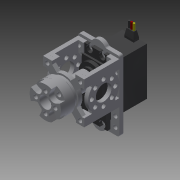
# Autodesk Inventor part: Servo with servo blocks
Saved by Autodesk Inventor 2013 (Build 170138000, 138)
## iProperties
Created: 2012-11-17
Part Number: Servo with servo blocks
Material: Generic
Document SubType Name: Modeling
Designer: niemitalo_dan
Density: 1 g/cm^3
Author: niemitalo_dan
Autodesk Inventor part; units mm, degrees
ref_plane "YZ Plane" through (0, 0, 0) normal (1, 0, 0) x (0, 1, 0)
ref_plane "XZ Plane" through (0, 0, 0) normal (0, 1, 0) x (-1, 0, 0)
sketch "Sketch1" plane through (0, 0, 0) normal (0, 0, 1) x (1, 0, 0)
  line L0 (-9.9314, 19.3675) -> (9.9314, 19.3675)
  line L1 (9.9314, 19.3675) -> (9.9314, -19.3675)
  line L2 (9.9314, -19.3675) -> (-9.9314, -19.3675)
  line L3 (-9.9314, -19.3675) -> (-9.9314, 19.3675)
  point P0 (0, 0)
  point P1 (-9.9314, 0)
  point P2 (0, 19.3675)
  dimension "d0" = 19.8628
  dimension "d1" = 38.735
  constraints: 8 end point, 2 midpoint, 2 parallel, 1 horizontal, 1 horizontal alignment, 1 perpendicular, 1 vertical alignment
  measures "d0" distance of L1.end L2.end
  measures "d1" distance of L0.end L1.end
extrude "Extrusion1" add sketch "Sketch1" along normal blind 33.147
sketch "Sketch2" plane through (0, 0, 33.147) normal (0, 0, 1) x (1, 0, 0)
  line L0 (9.9314, 19.3675) -> (-9.9314, 19.3675) projected
  line L1 (-9.9314, 19.3675) -> (-9.9314, -19.3675) projected
  line L2 (-9.9314, -19.3675) -> (9.9314, -19.3675) projected
  line L3 (-9.2964, 18.7325) -> (9.2964, 18.7325)
  line L4 (9.2964, 18.7325) -> (9.2964, -15.0495)
  line L5 (9.2964, -15.0495) -> (-9.2964, -15.0495)
  line L6 (-9.2964, -15.0495) -> (-9.2964, 18.7325)
  arc A0 (-3.6998, -15.0495) -> (3.6998, -15.0495) centre (0, -10.9617) ccw
  point P0 (0, 0)
  point P1 (0, 18.7325)
  dimension "d4" = 0.635
  dimension "d5" = 0.635
  dimension "d6" = 4.318
  constraints: 8 end point, 2 parallel, 2 point on circle, 2 point on line, 2 vertical alignment, 1 centre point, 1 horizontal, 1 midpoint, 1 perpendicular
  measures "d4" distance between parallel lines of L0 L3
  measures "d5" distance between parallel lines of L1 L6
  measures "d6" distance between parallel lines of L2 L5
extrude "Extrusion2" add sketch "Sketch2" along normal blind 2.794 contours L3 L4 L5 L6
sketch "Sketch3" plane through (0, 0, 35.941) normal (0, 0, 1) x (1, 0, 0)
  circle A0 centre (0, 9.4361) radius 6.4516
  line L0 (9.9314, 19.3675) -> (-9.9314, 19.3675) projected
  point P0 (0, 0)
  dimension "d9" = 12.9032
  dimension "d11" = 9.9314
  constraints: 1 centre point, 1 vertical alignment
  measures "d9" diameter of A0
  measures "d11" distance from line of L0 A0.centre
extrude "Extrusion3" add sketch "Sketch3" along normal blind 1.778
fillet "Fillet1" radius 9.2964 2 edges at (9.2964, 18.7325, 34.544) (-9.2964, 18.7325, 34.544)
ref_plane "Work Plane1" through (0, 0, 29.083) normal (0, 0, 1) x (1, 0, 0)
sketch "Sketch4" plane through (0, 0, 29.083) normal (0, 0, 1) x (1, 0, 0)
  line L0 (9.9314, 19.3675) -> (9.9314, -19.3675) projected
  line L1 (9.9314, -19.3675) -> (-9.9314, -19.3675) projected
  line L2 (-9.9314, -19.3675) -> (-9.9314, 19.3675) projected
  line L3 (-9.9314, 19.3675) -> (9.9314, 19.3675) projected
  line L4 (-9.3599, 19.3675) -> (9.3599, 19.3675)
  line L5 (9.3599, 19.3675) -> (9.3599, 26.4795)
  line L6 (-9.3599, 26.4795) -> (-9.3599, 19.3675)
  circle A0 centre (-5.1689, 23.9395) radius 2.667
  circle A1 centre (5.1689, 23.9395) radius 2.667
  line L7 (-5.9821, 26.4795) -> (-9.3599, 26.4795)
  line L8 (9.3599, 26.4795) -> (5.9821, 26.4795)
  line L9 (4.3557, 26.4795) -> (-4.3557, 26.4795)
  point P0 (0, 0)
  point P1 (0, 26.4795)
  dimension "d16" = 18.7198
  dimension "d18" = 7.112
  dimension "d20" = 5.334
  dimension "d21" = 4.191
  dimension "d22" = 4.191
  constraints: 12 end point, 4 parallel, 4 point on circle, 2 centre point, 1 equal radius, 1 horizontal, 1 horizontal alignment, 1 midpoint, 1 perpendicular, 1 point on line, 1 vertical alignment
  measures "d16" distance of L5.end L6.start
  measures "d18" distance of L6.start L4.start
  measures "d20" diameter of A0
  measures "d21" distance from line of L6 A0.centre
  measures "d22" distance from line of L5 A1.centre
extrude "Extrusion4" add sketch "Sketch4" along normal blind 2.54 contours L3 L6 L7 A0 L9 A1 L8 L5
fillet "Fillet2" radius 0.254 4 edges at (-5.9821, 26.4795, 30.353) (-4.3557, 26.4795, 30.353) (4.3557, 26.4795, 30.353) (5.9821, 26.4795, 30.353)
mirror "Mirror1" about plane through (0, 0, 0) normal (0, 1, 0) of "Extrusion4", "Fillet2"
sketch "Sketch5" plane through (-9.9314, 19.3675, 0) normal (0, 1, 0) x (1, 0, 0)
  line L0 (0, 0) -> (19.8628, 0) projected
  line L1 (6.1214, -0.254) -> (13.7414, -0.254)
  line L2 (13.7414, -0.254) -> (13.7414, -4.572)
  line L3 (13.7414, -4.572) -> (6.1214, -4.572)
  line L4 (6.1214, -4.572) -> (6.1214, -0.254)
  point P0 (9.9314, 0)
  point P1 (9.9314, -0.254)
  point P2 (9.9314, 0)
  dimension "d26" = 7.62
  dimension "d27" = 4.318
  dimension "d28" = 0.254
  constraints: 8 end point, 2 midpoint, 2 parallel, 1 horizontal, 1 perpendicular, 1 vertical alignment
  measures "d26" distance of L2.end L3.end
  measures "d27" distance of L1.end L2.end
  measures "d28" distance between parallel lines of L0 L1
extrude "Extrusion5" add sketch "Sketch5" along normal blind 1.5875
sketch "Sketch6" plane through (-9.9314, 20.955, 0) normal (0, 1, 0) x (1, 0, 0)
  line L0 (13.7414, -0.254) -> (6.1214, -0.254) projected
  line L1 (6.1214, -0.254) -> (6.1214, -4.572) projected
  line L2 (6.1214, -4.572) -> (13.7414, -4.572) projected
  line L3 (13.7414, -4.572) -> (13.7414, -0.254) projected
  point P0 (9.9314, 0)
extrude "Extrusion6" add sketch "Sketch6" along normal blind 5.08 draft -10
sketch "Sketch7" plane through (-9.9314, 26.035, 0) normal (0, 1, 0) x (1, 0, 0)
  circle A0 centre (9.9314, -2.413) radius 0.7937
  point P0 (9.9314, 0)
  dimension "d33" = 1.5875
  constraints: 1 centre point
  measures "d33" diameter of A0
extrude "Extrusion7" add sketch "Sketch7" along normal blind 5.08 separate body
sketch "Sketch8" plane through (-9.9314, 26.035, 0) normal (0, 1, 0) x (1, 0, 0)
  line L0 (7.0171, -3.6763) -> (7.0171, -1.1497) projected
  circle A0 centre (8.0331, -2.413) radius 0.7937
  point P0 (9.9314, 0)
  dimension "d36" = 1.5875
  dimension "d37" = 1.016
  constraints: 1 centre point
  measures "d36" diameter of A0
  measures "d37" distance from line of L0 A0.centre
extrude "Extrusion8" add sketch "Sketch8" along normal blind 5.08 bodies 1
sketch "Sketch9" plane through (-9.9314, 26.035, 0) normal (0, 1, 0) x (1, 0, 0)
  line L0 (12.8457, -1.1497) -> (12.8457, -3.6763) projected
  circle A0 centre (11.8297, -2.413) radius 0.7938
  point P0 (9.9314, 0)
  dimension "d40" = 1.5875
  dimension "d41" = 1.016
  constraints: 1 centre point
  measures "d40" diameter of A0
  measures "d41" distance from line of L0 A0.centre
extrude "Extrusion9" add sketch "Sketch9" along normal blind 5.08 separate body
sketch "Sketch10" plane through (0, 0, 29.083) normal (0, 0, -1) x (-1, 0, 0)
  line L0 (-9.9314, -19.3675) -> (-9.9314, 19.3675) construction
  line L1 (-9.9314, 19.3675) -> (-9.3599, 19.3675) construction
  line L2 (-9.3599, 19.3675) -> (-9.3599, 26.4795) construction
  line L3 (-9.3599, 26.4795) -> (-6.9873, 26.4795) construction
  arc A0 (-6.8291, 26.0267) -> (-6.9873, 26.4795) centre (-6.9873, 26.2255) ccw construction
  arc A1 (-6.8291, 26.0267) -> (-3.5087, 26.0267) centre (-5.1689, 23.9395) ccw construction
  arc A2 (-3.3505, 26.4795) -> (-3.5087, 26.0267) centre (-3.3505, 26.2255) ccw construction
  line L4 (-3.3505, 26.4795) -> (3.3505, 26.4795) construction
  arc A3 (3.5087, 26.0267) -> (3.3505, 26.4795) centre (3.3505, 26.2255) ccw construction
  arc A4 (3.5087, 26.0267) -> (6.8291, 26.0267) centre (5.1689, 23.9395) ccw construction
  arc A5 (6.9873, 26.4795) -> (6.8291, 26.0267) centre (6.9873, 26.2255) ccw construction
  line L5 (6.9873, 26.4795) -> (9.3599, 26.4795) construction
  line L6 (9.3599, 26.4795) -> (9.3599, 19.3675) construction
  line L7 (9.3599, 19.3675) -> (9.9314, 19.3675) construction
  line L8 (9.9314, 19.3675) -> (9.9314, -19.3675) construction
  line L9 (9.9314, -19.3675) -> (9.3599, -19.3675) construction
  line L10 (9.3599, -19.3675) -> (-9.3599, -19.3675) construction
  line L11 (-9.3599, -19.3675) -> (-9.9314, -19.3675) construction
  line L12 (-9.3599, 19.3675) -> (9.3599, 19.3675) construction
  line L13 (9.3599, -19.3675) -> (9.3599, -26.4795) construction
  line L14 (9.3599, -26.4795) -> (6.9873, -26.4795) construction
  arc A6 (6.8291, -26.0267) -> (6.9873, -26.4795) centre (6.9873, -26.2255) ccw construction
  arc A7 (6.8291, -26.0267) -> (3.5087, -26.0267) centre (5.1689, -23.9395) ccw construction
  arc A8 (3.3505, -26.4795) -> (3.5087, -26.0267) centre (3.3505, -26.2255) ccw construction
  line L15 (3.3505, -26.4795) -> (-3.3505, -26.4795) construction
  arc A9 (-3.5087, -26.0267) -> (-3.3505, -26.4795) centre (-3.3505, -26.2255) ccw construction
  arc A10 (-3.5087, -26.0267) -> (-6.8291, -26.0267) centre (-5.1689, -23.9395) ccw construction
  arc A11 (-6.9873, -26.4795) -> (-6.8291, -26.0267) centre (-6.9873, -26.2255) ccw construction
  line L16 (-6.9873, -26.4795) -> (-9.3599, -26.4795) construction
  line L17 (-9.3599, -26.4795) -> (-9.3599, -19.3675) construction
  line L18 (-16.6688, 28.575) -> (16.6687, 28.575)
  line L19 (16.6687, 28.575) -> (16.6688, -28.575)
  line L20 (16.6688, -28.575) -> (-16.6687, -28.575)
  line L21 (-16.6687, -28.575) -> (-16.6688, 28.575)
  line L22 (-9.9314, 19.3675) -> (9.9314, 19.3675)
  line L23 (9.9314, 19.3675) -> (9.9314, -19.3675)
  line L24 (9.9314, -19.3675) -> (-9.9314, -19.3675)
  line L25 (-9.9314, -19.3675) -> (-9.9314, 19.3675)
  circle A12 centre (-5.1689, 23.9395) radius 1.7272
  circle A13 centre (5.1689, 23.9395) radius 1.7272
  circle A14 centre (-5.1689, -23.9395) radius 1.7272
  circle A15 centre (5.1689, -23.9395) radius 1.7272
  circle A16 centre (-13.3033, 23.075) radius 1.7272
  arc A17 (5.4993, 28.575) -> (-5.4993, 28.575) centre (0, 25.4) ccw
  line L26 (-21.6347, 31.75) -> (28.9033, 31.75) construction
  arc A18 (-5.4993, -28.575) -> (5.4993, -28.575) centre (0, -25.4) ccw
  line L27 (-14.4215, -31.75) -> (20.7079, -31.75) construction
  circle A19 centre (13.3033, 23.075) radius 1.7272
  circle A20 centre (-13.3033, 15.1375) radius 1.7272
  circle A21 centre (-13.3033, 4.0885) radius 1.7272
  circle A22 centre (13.3032, 15.1375) radius 1.7272
  circle A23 centre (13.3032, 4.0885) radius 1.7272
  line L28 (-16.6688, 0) -> (16.6688, 0) construction
  circle A24 centre (-13.3033, -23.075) radius 1.7272
  circle A25 centre (13.3033, -23.075) radius 1.7272
  circle A26 centre (-13.3033, -15.1375) radius 1.7272
  circle A27 centre (-13.3033, -4.0885) radius 1.7272
  circle A28 centre (13.3032, -15.1375) radius 1.7272
  circle A29 centre (13.3032, -4.0885) radius 1.7272
  point P0 (0, 0)
  point P1 (0, 28.575)
  dimension "d44" = 3.4544
  dimension "d47" = 57.15
  dimension "d48" = 3.175
  dimension "d49" = 6.35
  dimension "d50" = 6.35
  dimension "d51" = 3.175
  dimension "d52" = 5.5
  dimension "d53" = 3.3655
  dimension "d54" = 3.3655
  dimension "d55" = 33.3375
  dimension "d56" = 7.9375
  dimension "d57" = 11.049
  constraints: 22 end point, 18 centre point, 9 equal radius, 7 vertical alignment, 6 symmetric about line, 5 parallel, 4 coincident, 4 horizontal alignment, 4 point on circle, 4 point on line, 3 midpoint, 3 perpendicular, 2 horizontal, 2 tangent, 6 other
  measures "d44" diameter of A12
  measures "d47" distance of L20.end L18.start
  measures "d48" distance between parallel lines of L18 L26
  measures "d49" radius of A17
  measures "d50" radius of A18
  measures "d51" distance between parallel lines of L20 L27
  measures "d52" distance from line of L18 A16.centre
  measures "d53" distance from line of L21 A16.centre
  measures "d54" distance from line of L19 A19.centre
  measures "d55" distance of L19.end L20.end
  measures "d56" distance of A16.centre A20.centre
  measures "d57" distance of A20.centre A21.centre
extrude "Extrusion10" add sketch "Sketch10" along normal blind 3.175 separate body
fillet "Fillet3" radius 1.5875 8 edges at (-16.6687, 28.575, 27.4955) (-16.6688, -28.575, 27.4955) (-5.4993, -28.575, 27.4955) (5.4993, -28.575, 27.4955) (16.6687, -28.575, 27.4955) (5.4993, 28.575, 27.4955) (16.6688, 28.575, 27.4955) (-5.4993, 28.575, 27.4955)
sketch "Sketch11" plane through (0, 9.4361, 37.719) normal (0, 0, 1) x (1, 0, 0)
  circle A0 centre (0, 0) radius 6.4516 projected
  circle A1 centre (0, 0) radius 1.5875
  point P0 (0, -9.4361)
  dimension "d61" = 3.175
  constraints: 1 centre point, 1 coincident
  measures "d61" diameter of A1
extrude "Extrusion11" add sketch "Sketch11" along normal blind 1.5875 separate body contours A1
sketch "Sketch12" plane through (0, 0, 29.083) normal (0, 0, 1) x (1, 0, 0)
  line L0 (-9.9314, -19.3675) -> (-9.9314, 19.3675) projected
  line L1 (-9.9314, 19.3675) -> (9.9314, 19.3675) projected
  line L2 (9.9314, 19.3675) -> (9.9314, -19.3675) projected
  circle A0 centre (-13.3032, -4.0885) radius 1.7272 projected
  circle A1 centre (13.3033, -4.0885) radius 1.7272 projected
  circle A2 centre (-13.3033, 23.075) radius 1.7272 projected
  circle A3 centre (13.3033, 23.075) radius 1.7272 projected
  line L3 (6.35, 28.575) -> (15.0813, 28.575) projected
  line L4 (-15.0812, 28.575) -> (-6.35, 28.575) projected
  line L5 (-16.6688, -26.9875) -> (-16.6687, 26.9875) projected
  line L6 (16.6688, 26.9875) -> (16.6687, -26.9875) projected
  line L7 (-16.6687, 26.4668) -> (-9.3918, 26.4668)
  line L8 (-9.3918, 26.4668) -> (-9.3918, 19.3675)
  line L9 (-9.3918, 19.3675) -> (-16.6687, 19.3675)
  line L10 (-16.6687, 19.3675) -> (-16.6687, 26.4668)
  line L11 (-16.6688, -0.9135) -> (-9.9314, -0.9135)
  line L12 (-9.9314, -0.9135) -> (-9.9314, -7.2635)
  line L13 (-9.9314, -7.2635) -> (-16.6688, -7.2635)
  line L14 (-16.6688, -7.2635) -> (-16.6688, -0.9135)
  line L15 (16.6688, -0.9135) -> (9.9314, -0.9135)
  line L16 (9.9314, -0.9135) -> (9.9314, -7.2635)
  line L17 (9.9314, -7.2635) -> (16.6688, -7.2635)
  line L18 (16.6688, -7.2635) -> (16.6688, -0.9135)
  line L19 (9.3087, 19.3675) -> (16.6688, 19.3675)
  line L20 (16.6688, 19.3675) -> (16.6688, 26.4668)
  line L21 (16.6688, 26.4668) -> (9.3087, 26.4668)
  line L22 (9.3087, 26.4668) -> (9.3087, 19.3675)
  point P0 (0, 0)
  dimension "d66" = 2.1082
  dimension "d67" = 2.1082
  dimension "d68" = 3.175
  dimension "d69" = 3.175
  constraints: 32 end point, 8 parallel, 8 point on line, 4 horizontal, 4 perpendicular, 2 collinear
  measures "d66" distance between parallel lines of L4 L7
  measures "d67" distance between parallel lines of L3 L21
  measures "d68" distance from line of L11 A0.centre
  measures "d69" distance from line of L13 A0.centre
extrude "Extrusion12" add sketch "Sketch12" along normal blind 3.175 separate body contours L13 L5 L11 L0 | L9 L5 L7 L8 L1
sketch "Sketch13" plane through (0, 0, 32.258) normal (0, 0, 1) x (1, 0, 0)
  line L0 (-16.6687, 26.4668) -> (-13.4937, 26.4668)
  line L1 (-13.4937, 26.4668) -> (-13.4937, -7.2635)
  line L2 (-13.4937, -7.2635) -> (-16.6687, -7.2635)
  line L3 (-16.6687, -7.2635) -> (-16.6687, 26.4668)
  line L4 (9.9314, 19.3675) -> (9.9314, -19.3675) projected
  line L5 (9.9314, -19.3675) -> (-9.9314, -19.3675) projected
  line L6 (-9.9314, -19.3675) -> (-9.9314, 19.3675) projected
  line L7 (-9.9314, 19.3675) -> (9.9314, 19.3675) projected
  circle A0 centre (-13.3033, 23.075) radius 1.7272 projected
  line L8 (-9.3918, 19.3675) -> (-16.6687, 19.3675) projected
  line L9 (-16.6687, 19.3675) -> (-16.6687, 26.4668) projected
  line L10 (-16.6687, 26.4668) -> (-9.3918, 26.4668) projected
  line L11 (-9.3918, 26.4668) -> (-9.3918, 19.3675) projected
  circle A1 centre (-13.3032, -4.0885) radius 1.7272 projected
  line L12 (-16.6688, -0.9135) -> (-9.9314, -0.9135) projected
  line L13 (-9.9314, -0.9135) -> (-9.9314, -7.2635) projected
  line L14 (-9.9314, -7.2635) -> (-16.6688, -7.2635) projected
  line L15 (-16.6688, -7.2635) -> (-16.6688, -0.9135) projected
  line L16 (-16.6688, -7.2635) -> (-9.9314, -7.2635) projected
  point P0 (0, 0)
  dimension "d72" = 3.175
  constraints: 8 end point, 2 parallel, 1 collinear, 1 horizontal, 1 perpendicular
  measures "d72" distance of L1.end L2.end
extrude "Extrusion13" add sketch "Sketch13" along normal blind 19.05 contours L0 L1 A0 L8 L3 | L8 L1 L12 L3 | L1 A0 | L12 L1 A1 L2 L3 | L1 A1 picked at (-13.6297, 22.5349) picked at (-13.989, -3.9498) bodies 6
sketch "Sketch14" plane through (0, 0, 51.308) normal (0, 0, 1) x (1, 0, 0)
  line L0 (-13.4937, 26.4668) -> (-13.4937, 24.7917) construction
  arc A0 (-13.4937, 21.3583) -> (-13.4937, 24.7917) centre (-13.3033, 23.075) ccw construction
  line L1 (-13.4937, 21.3583) -> (-13.4937, 19.3675) construction
  line L2 (-13.4937, 19.3675) -> (-9.3918, 19.3675) construction
  line L3 (-9.3918, 19.3675) -> (-9.3918, 26.4668) construction
  line L4 (-9.3918, 26.4668) -> (-13.4937, 26.4668) construction
  line L5 (-13.4937, -0.9135) -> (-13.4937, -2.3718) construction
  arc A1 (-13.4937, -5.8052) -> (-13.4937, -2.3718) centre (-13.3032, -4.0885) ccw construction
  line L6 (-13.4937, -5.8052) -> (-13.4937, -7.2635) construction
  line L7 (-13.4937, -7.2635) -> (-9.9314, -7.2635) construction
  line L8 (-9.9314, -7.2635) -> (-9.9314, -0.9135) construction
  line L9 (-9.9314, -0.9135) -> (-13.4937, -0.9135) construction
  line L10 (-16.6687, 19.3675) -> (-13.4937, 19.3675) construction
  line L11 (-13.4937, -0.9135) -> (-16.6688, -0.9135) construction
  circle A2 centre (-13.3033, 23.075) radius 1.7272 construction
  circle A3 centre (-13.3032, -4.0885) radius 1.7272 construction
  line L12 (-16.6687, 26.4668) -> (-9.3918, 26.4668)
  line L13 (-9.3918, 26.4668) -> (-9.3918, 19.3675)
  line L14 (-9.3918, 19.3675) -> (-16.6687, 19.3675)
  line L15 (-16.6687, 19.3675) -> (-16.6687, 26.4668)
  line L16 (-16.6688, -0.9135) -> (-9.9314, -0.9135)
  line L17 (-9.9314, -0.9135) -> (-9.9314, -7.2635)
  line L18 (-9.9314, -7.2635) -> (-16.6688, -7.2635)
  line L19 (-16.6688, -7.2635) -> (-16.6688, -0.9135)
  circle A4 centre (-13.3032, -4.0885) radius 1.7272
  circle A5 centre (-13.3033, 23.075) radius 1.7272
  point P0 (0, 0)
  constraints: 16 end point, 4 parallel, 2 centre point, 2 coincident, 2 horizontal, 2 perpendicular, 1 concentric
extrude "Extrusion14" add sketch "Sketch14" along normal blind 3.175 bodies 6
sketch "Sketch16" plane through (-16.6688, 19.3675, 29.083) normal (-1, 0, 0) x (0, 0, 1)
  line L0 (22.225, 0) -> (22.225, -20.281) projected
  line L1 (0, 7.0993) -> (25.4, 7.0993) projected
  line L2 (3.175, 0) -> (3.175, -20.281) projected
  circle A0 centre (12.7, -10.1405) radius 12.7
  line L3 (3.175, -1.7402) -> (3.175, -18.5408)
  line L4 (22.225, -1.7402) -> (22.225, -18.5408)
  point P0 (-29.083, -19.3675)
  point P1 (12.7, 7.0993)
  point P2 (22.225, -10.1405)
  dimension "d80" = 25.4
  constraints: 4 end point, 4 point on circle, 4 point on line, 2 midpoint, 1 centre point, 1 horizontal alignment, 1 vertical alignment
  measures "d80" diameter of A0
extrude "Extrusion15" add sketch "Sketch16" against normal blind 3.175 contours A0 L0 | L2 A0 bodies 6
sketch "Sketch17" plane through (-16.6688, 19.3675, 29.083) normal (-1, 0, 0) x (0, 0, 1)
  arc A0 (22.225, -18.5408) -> (22.225, -1.7402) centre (12.7, -10.1405) ccw construction
  arc A1 (3.175, -1.7402) -> (3.175, -18.5408) centre (12.7, -10.1405) ccw construction
  circle A2 centre (12.7, -10.1405) radius 6.35
  circle A3 centre (12.7, -10.1405) radius 9.525 construction
  circle A4 centre (12.7, -0.6155) radius 1.7272
  circle A5 centre (5.9648, -3.4053) radius 1.7272
  circle A6 centre (3.175, -10.1405) radius 1.7272
  circle A7 centre (5.9648, -16.8757) radius 1.7272
  circle A8 centre (12.7, -19.6655) radius 1.7272
  circle A9 centre (19.4352, -16.8757) radius 1.7272
  circle A10 centre (22.225, -10.1405) radius 1.7272
  circle A11 centre (19.4352, -3.4053) radius 1.7272
  point P0 (-29.083, -19.3675)
  dimension "d85" = 19.05
  dimension "d84" = 12.7
  dimension "d86" = 3.4544
  dimension "d89" = 360
  constraints: 9 centre point, 2 coincident, 2 vertical alignment, 19 other
  measures "d84" diameter of A2
  measures "d86" diameter of A4
extrude "Extrusion16" cut sketch "Sketch17" against normal blind 3.175 bodies 6
mirror "Mirror2" about plane through (0, 0, 0) normal (1, 0, 0) bodies 6
sketch "Sketch18" plane through (0, 0, 54.483) normal (0, 0, 1) x (1, 0, 0)
  circle A0 centre (-13.3033, 23.075) radius 1.7272 projected
  line L0 (-16.6687, 19.3675) -> (-9.3918, 19.3675) projected
  line L1 (-9.3918, 19.3675) -> (-9.3918, 26.4668) projected
  circle A1 centre (-13.3032, -4.0885) radius 1.7272 projected
  line L2 (-9.9314, -7.2635) -> (-9.9314, -0.9135) projected
  line L3 (-9.9314, -0.9135) -> (-16.6688, -0.9135) projected
  line L4 (-16.6688, -0.9135) -> (-16.6688, -7.2635) projected
  line L5 (-16.6688, -7.2635) -> (-9.9314, -7.2635) projected
  circle A2 centre (13.3033, 23.075) radius 1.7272 projected
  line L6 (9.3918, 26.4668) -> (16.6687, 26.4668) projected
  line L7 (9.3918, 19.3675) -> (9.3918, 26.4668) projected
  line L8 (16.6687, 19.3675) -> (9.3918, 19.3675) projected
  line L9 (16.6687, 26.4668) -> (16.6687, 19.3675) projected
  circle A3 centre (13.3032, -4.0885) radius 1.7272 projected
  line L10 (9.9314, -7.2635) -> (9.9314, -0.9135) projected
  line L11 (16.6688, -7.2635) -> (9.9314, -7.2635) projected
  line L12 (16.6688, -0.9135) -> (16.6688, -7.2635) projected
  line L13 (9.9314, -0.9135) -> (16.6688, -0.9135) projected
  circle A4 centre (0, 9.4361) radius 6.4516 projected
  circle A5 centre (0, 9.4361) radius 12.065
  line L14 (-14.2655, 19.3675) -> (-10.4185, 15.5205)
  line L15 (-9.3918, 23.8332) -> (-5.6532, 20.0947)
  line L16 (-9.9314, -7.2635) -> (-9.9314, -0.9135) projected
  line L17 (-9.9314, -0.9135) -> (-16.6688, -0.9135) projected
  circle A6 centre (-13.3033, 23.075) radius 1.7272 projected
  line L18 (-9.3918, 26.4668) -> (-16.6687, 26.4668) projected
  line L19 (-16.6687, 26.4668) -> (-16.6687, 19.3675) projected
  line L20 (-16.6687, 19.3675) -> (-9.3918, 19.3675) projected
  line L21 (-9.3918, 19.3675) -> (-9.3918, 26.4668) projected
  line L22 (-14.798, -0.9135) -> (-10.4604, 3.4241)
  line L23 (-9.9314, -5.3864) -> (-5.7277, -1.1827)
  line L24 (-9.9314, 19.3675) -> (-9.9314, -19.3675) projected
  line L25 (0, 9.4361) -> (0, 21.5011) construction
  line L26 (14.2655, 19.3675) -> (10.4185, 15.5205)
  line L27 (9.3918, 23.8332) -> (5.6532, 20.0947)
  line L28 (14.798, -0.9135) -> (10.4604, 3.4241)
  line L29 (9.9314, -5.3864) -> (5.7277, -1.1827)
  arc A7 (10.4185, 15.5205) -> (5.6532, 20.0947) centre (0, 9.4361) ccw
  arc A8 (5.7277, -1.1827) -> (10.4604, 3.4241) centre (0, 9.4361) ccw
  line L30 (9.9314, -5.3864) -> (9.9314, -0.9135)
  line L31 (14.798, -0.9135) -> (9.9314, -0.9135)
  line L32 (14.2655, 19.3675) -> (9.3918, 19.3675)
  line L33 (9.3918, 19.3675) -> (9.3918, 23.8332)
  point P0 (0, 0)
  dimension "d93" = 24.13
  dimension "d94" = 45
  dimension "d96" = 6.604
  dimension "d97" = 3.302
  dimension "d100" = 45
  dimension "d101" = 3.302
  dimension "d102" = 6.604
  constraints: 26 end point, 9 point on circle, 8 symmetric about line, 4 collinear, 4 point on line, 3 centre point, 3 coincident, 3 parallel
  measures "d93" diameter of A5
  measures "d94" angle of L0 L14
  measures "d96" distance between parallel lines of L15 L14
  measures "d97" distance from line of A0.centre L15
  measures "d100" angle of L24 L22
  measures "d101" distance from line of A1.centre L22
  measures "d102" distance between parallel lines of L23 L22
extrude "Extrusion18" add sketch "Sketch18" along normal blind 3.175 separate body
sketch "Sketch19" plane through (0, 0, 57.658) normal (0, 0, 1) x (1, 0, 0)
  circle A0 centre (0, 9.4361) radius 6.4516 projected
  arc A1 (10.4604, 3.4241) -> (10.4185, 15.5205) centre (0, 9.4361) ccw projected
  circle A2 centre (0, 9.4361) radius 10.7315
  point P0 (0, 0)
  dimension "d105" = 21.463
  constraints: 1 centre point, 1 coincident
  measures "d105" diameter of A2
extrude "Extrusion19" add sketch "Sketch19" along normal blind 1.8288 bodies 7
sketch "Sketch20" plane through (0, 9.4361, 39.3065) normal (0, 0, 1) x (1, 0, 0)
  circle A0 centre (0, 0) radius 1.5875 construction
  circle A1 centre (0, 0) radius 6.35
  point P0 (0, -9.4361)
  dimension "d108" = 12.7
  constraints: 1 centre point, 1 coincident
  measures "d108" diameter of A1
extrude "Extrusion20" add sketch "Sketch20" along normal blind 21.7805 separate body
sketch "Sketch21" plane through (0, 9.4361, 61.087) normal (0, 0, 1) x (1, 0, 0)
  circle A0 centre (0, 0) radius 6.35 construction
  circle A1 centre (0, 0) radius 12.7
  circle A2 centre (0, 0) radius 9.525 construction
  circle A3 centre (0, 9.525) radius 1.7272
  circle A4 centre (-6.7352, 6.7352) radius 1.7272
  circle A5 centre (-9.525, 0) radius 1.7272
  circle A6 centre (-6.7352, -6.7352) radius 1.7272
  circle A7 centre (0, -9.525) radius 1.7272
  circle A8 centre (6.7352, -6.7352) radius 1.7272
  circle A9 centre (9.525, 0) radius 1.7272
  circle A10 centre (6.7352, 6.7352) radius 1.7272
  point P0 (0, -9.4361)
  dimension "d112" = 19.05
  dimension "d111" = 25.4
  dimension "d113" = 3.4544
  dimension "d116" = 360
  constraints: 9 centre point, 2 coincident, 2 vertical alignment, 19 other
  measures "d111" diameter of A1
  measures "d113" diameter of A3
extrude "Extrusion21" add sketch "Sketch21" along normal blind 5.08 bodies 8
sketch "Sketch22" plane through (0, 9.4361, 66.167) normal (0, 0, 1) x (1, 0, 0)
  circle A0 centre (0, 0) radius 12.7 construction
  circle A1 centre (0, 0) radius 3.81
  point P0 (0, -9.4361)
  dimension "d120" = 7.62
  constraints: 1 centre point, 1 coincident
  measures "d120" diameter of A1
extrude "Extrusion22" cut sketch "Sketch22" against normal up to surface (26.8605 mm away) bodies 8
sketch "Sketch23" plane through (0, 9.4361, 66.167) normal (0, 0, 1) x (1, 0, 0)
  circle A0 centre (0, 0) radius 3.81 construction
  circle A1 centre (6.7352, 6.7352) radius 1.7272 projected
  circle A2 centre (6.7352, -6.7352) radius 1.7272 projected
  circle A3 centre (-6.7352, -6.7352) radius 1.7272 projected
  circle A4 centre (-6.7352, 6.7352) radius 1.7272 projected
  circle A5 centre (0, 0) radius 12.7 projected
  circle A6 centre (0, 0) radius 4.7625
  circle A7 centre (0, 0) radius 7.9375 construction
  circle A8 centre (0, 7.9375) radius 1.7272
  circle A9 centre (-7.9375, 0) radius 1.7272
  circle A10 centre (0, -7.9375) radius 1.7272
  circle A11 centre (7.9375, 0) radius 1.7272
  point P0 (0, -9.4361)
  dimension "d124" = 15.875
  dimension "d123" = 9.525
  dimension "d125" = 3.4544
  dimension "d128" = 360
  constraints: 5 centre point, 2 coincident, 2 vertical alignment, 11 other
  measures "d123" diameter of A6
  measures "d125" diameter of A8
extrude "Extrusion23" add sketch "Sketch23" along normal blind 6.35 separate body
sketch "Sketch24" plane through (0, 9.4361, 72.517) normal (0, 0, 1) x (1, 0, 0)
  circle A0 centre (-6.7352, 6.7352) radius 1.7272 construction
  circle A1 centre (0, 0) radius 12.7 construction
  arc A2 (-8.3246, 3.3266) -> (-3.3266, 8.3246) centre (-6.7352, 6.7352) ccw
  arc A3 (-4.907, 11.7137) -> (-11.7137, 4.907) centre (0, 0) ccw
  line L0 (-3.3266, 8.3246) -> (-4.907, 11.7137)
  line L1 (-8.3246, 3.3266) -> (-11.7137, 4.907)
  line L2 (-6.7352, 6.7352) -> (0, 0) construction
  point P0 (0, -9.4361)
  dimension "d133" = 20
  dimension "d134" = 20
  constraints: 6 end point, 4 point on circle, 2 centre point, 2 coincident, 2 tangent, 3 other
  measures "d133" angle of L0 L2
  measures "d134" angle of L2 L1
extrude "Extrusion24" cut sketch "Sketch24" against normal blind 4.2672 bodies 9
pattern_circular "Circular Pattern1" count 4 over 360 about axis through (0, 9.4361, 66.167) along (0, 0, 1) of "Extrusion24" bodies 9
equation "\"d5\" = d4"
equation "\"d22\" = d21"
equation "\"d54\" = d53"
equation "\"d97\" = 0.5 * d96"
